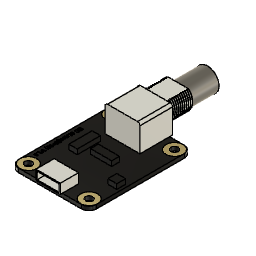
Device-pH-NodeController v5 (Autodesk Fusion 360 archive; units mm, degrees)
design "EC MEter DF Robot v1"
Autodesk Fusion 360 part; units mm, degrees
sketch "Sketch1" plane through (0, 0, 0) normal (0, 0, 1) x (1, 0, 0)
  line L0 (-7.7444, 8.9203) -> (6.5556, 8.9203)
  line L1 (6.5556, 8.9203) -> (6.5556, -4.4842)
  line L2 (6.5556, -4.4842) -> (-7.7444, -4.4842)
  line L3 (-7.7444, -4.4842) -> (-7.7444, 8.9203)
  line L4 (-16.3954, 7.7118) -> (15.6046, 7.7118)
  line L5 (15.6046, 7.7118) -> (15.6046, -34.4882)
  line L6 (15.6046, -34.4882) -> (-16.3954, -34.4882)
  line L7 (-16.3954, -34.4882) -> (-16.3954, 7.7118)
  line L8 (-5.3642, -27.7927) -> (4.6358, -27.7927)
  line L9 (4.6358, -27.7927) -> (4.6358, -35.2927)
  line L10 (4.6358, -35.2927) -> (-5.3642, -35.2927)
  line L11 (-5.3642, -35.2927) -> (-5.3642, -27.7927)
  circle A0 centre (-12.8954, 4.2118) radius 1.5
  circle A1 centre (-12.8954, 4.2118) radius 3.5
  circle A2 centre (12.1046, 4.2118) radius 3.5
  circle A3 centre (12.1046, 4.2118) radius 1.5
  circle A4 centre (-12.8954, -30.8882) radius 3.5
  circle A5 centre (-12.8954, -30.8882) radius 1.5
  circle A6 centre (12.1046, -30.8882) radius 3.5
  circle A7 centre (12.1046, -30.8882) radius 1.5
  line L12 (-9.5014, -8.0872) -> (-6.0322, -8.0872)
  line L13 (-6.0322, -8.0872) -> (-6.0322, -17.64)
  line L14 (-6.0322, -17.64) -> (-9.5014, -17.64)
  line L15 (-9.5014, -17.64) -> (-9.5014, -8.0872)
  line L16 (-3.468, -11.5563) -> (5.2301, -11.5563)
  line L17 (5.2301, -11.5563) -> (5.2301, -14.7741)
  line L18 (5.2301, -14.7741) -> (-3.468, -14.7741)
  line L19 (-3.468, -14.7741) -> (-3.468, -11.5563)
  line L20 (10.7856, -18.2306) -> (14.4434, -18.2306)
  line L21 (14.4434, -18.2306) -> (14.4434, -21.8884)
  line L22 (14.4434, -21.8884) -> (10.7856, -21.8884)
  line L23 (10.7856, -21.8884) -> (10.7856, -18.2306)
  line L24 (-15.6535, -7.3303) -> (-15.6535, -26.5939) construction
  line L25 (-15.6535, -26.5939) -> (-13.6535, -26.5939) construction
  line L26 (-13.6535, -26.5939) -> (-13.6535, -7.3303) construction
  line L27 (-13.6535, -7.3303) -> (-15.6535, -7.3303) construction
  dimension "d1" = 32
  dimension "d2" = 14.3
  dimension "d3" = 10
  dimension "d4" = 7.5
  dimension "d5" = 42.2
  dimension "d6" = 3
  dimension "d7" = 2
  dimension "d10" = 25
  dimension "d11" = -35.1
  text T0 "EC Meter(K=10) V1.0" font "Arial" height 2 bold align ink ink in box 0 x 0 at (-15.6535, -7.3303) x (0, -1) y (1, 0) spacing 1 height is em
  constraint horizontal L0
  constraint vertical L1
  constraint horizontal L2
  constraint vertical L3
  constraint horizontal L4
  constraint vertical L5
  constraint horizontal L6
  constraint vertical L7
  constraint horizontal L8
  constraint vertical L9
  constraint horizontal L10
  constraint vertical L11
  constraint tangent L4 A1
  constraint tangent L7 A1
  constraint horizontal L12
  constraint vertical L13
  constraint horizontal L14
  constraint vertical L15
  constraint horizontal L16
  constraint vertical L17
  constraint horizontal L18
  constraint vertical L19
  constraint horizontal L20
  constraint vertical L21
  constraint horizontal L22
  constraint vertical L23
  constraint perpendicular L24 L25
  constraint parallel L24 L26
  constraint parallel L25 L27
  measures "d1" distance of L4.start L4.end
  measures "d2" distance of L1.end L2.end
  measures "d3" distance of L8.start L8.end
  measures "d4" distance of L8.start L10.end
  measures "d5" distance of L4.start L6.end
  measures "d6" diameter of A0
extrude "Extrude1" add sketch "Sketch1" along normal blind 1.6 contours L1 L2 L3 L4 | A4 | A6 | L1 L2 L3 L4 L5 L6 L7 L8 L9 L11 A1 A2 | L4 L7 A1 | A1 | L4 L5 A2 | A2 | L6 L8 L9 L11 | A0 | A3 | A5 | A7 | L12 L13 L14 L15 | L16 L17 L18 L19 | L20 L21 L22 L23 makes body 1
extrude "Extrude2" cut sketch "Sketch1" along normal through all contours A0 | A3 | A5 | A7 bodies 1
extrude "Extrude3" add sketch "Sketch1" along normal blind 0.01 from surface at 1.6 contours A4 | A6 | A1 | A2 bodies 1
extrude "Extrude4" add sketch "Sketch1" along normal blind 11 from surface at 1.6 separate body contours L0 L1 L3 L4 | L1 L2 L3 L4 makes body 2
extrude "Extrude5" add sketch "Sketch1" along normal blind 4 from surface at 1.6 separate body contours L6 L8 L9 L11 | L6 L9 L10 L11 makes body 3
extrude "Extrude6" add sketch "Sketch1" along normal blind 2 from surface at 1.6 contours L12 L13 L14 L15 | L16 L17 L18 L19 | L20 L21 L22 L23 bodies 2 1
shell "Shell1" thickness 0.5 removed faces 1 at (1.3024, -35.2927, 2.9333) on bodies 3
sketch "Sketch2" plane through (0, 8.9203, 0) normal (0, 1, 0) x (-1, 0, 0)
  line L0 (-6.5556, 1.6) -> (7.7444, 1.6)
  line L1 (7.7444, 1.6) -> (7.7444, 12.6)
  line L2 (7.7444, 12.6) -> (-6.5556, 12.6)
  line L3 (-6.5556, 12.6) -> (-6.5556, 1.6)
  arc A0 (-4.0966, 11.8409) -> (5.2854, 11.8409) centre (0.5944, 8.1) ccw
  line L4 (-4.0966, 11.8409) -> (5.2854, 11.8409)
  circle A1 centre (0.5944, 7.117) radius 4.75
  circle A2 centre (0.5944, 7.117) radius 4.55
  circle A3 centre (0.5944, 7.117) radius 2
  circle A4 centre (0.5944, 7.117) radius 0.5
  dimension "d28" = 12
  dimension "d31" = 9.5
  dimension "d32" = -0.2
  dimension "d36" = 4
  dimension "d37" = 1
  constraint perpendicular L1 L4
  constraint concentric A1 A3
  constraint concentric A1 A4
  measures "d28" diameter of A0
  measures "d31" diameter of A1
  measures "d36" diameter of A3
  measures "d37" diameter of A4
extrude "Extrude7" add sketch "Sketch2" along normal blind 9.5 contours A0 L4 A1 | L4 A1 | A2 | A3 | A4 picked at (-0.0222, 11.6827) bodies 1 2
thread "Thread1" "AFBMA Standard Locknuts 0.469 N 01 3A" major diameter 11.844 minor diameter 10.9398 pitch 0.7937 angle 60 modelled right hand crest width 0.1197 on face at (-5.9336, 15.2536, 10.8373) crest through (4.0356, 8.7218, 11.7923) on bodies 2
extrude "Extrude8" add sketch "Sketch2" along normal blind 12 from surface at 9.5 separate body contours L4 A1 | L4 A1 makes body 4
extrude "Extrude9" add sketch "Sketch2" along normal blind 8.5 from surface at 9.5 separate body contours A3 makes body 5
extrude "Extrude10" add sketch "Sketch2" along normal blind 8.5 from surface at 9.5 separate body contours A4 makes body 6
fillet "Fillet1" radius 1 2 edges at (-7.7444, 2.218, 12.6) (6.5556, 2.218, 12.6) on bodies 2
fillet "Fillet2" radius 0.2 1 edges at (1.2703, 26.9203, 6.3938) on bodies 5
fillet "Fillet3" radius 3 4 edges at (15.6046, 7.7118, 0.8) (-16.3954, 7.7118, 0.8) (15.6046, -34.4882, 0.8) (-16.3954, -34.4882, 0.8) on bodies 1
extrude "Extrude11" add sketch "Sketch1" along normal blind 0.01 from surface at 1.6 text T0 bodies 1
